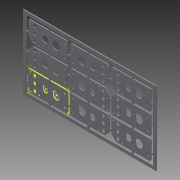
# Autodesk Inventor part: Granny Gearbox Output Plate Routing Template (9-up)
Saved by Autodesk Inventor 2015 (Build 190159000, 159)
## iProperties
Created: 2016-02-25
Part Number: Granny Gearbox Output Plate Routing Template (9-up)
Material: Generic
Document SubType Name: Modeling
Designer: sethbattis
Density: 1 g/cm^3
Appearance: Default
Author: sethbattis
Autodesk Inventor part; units mm, degrees
ref_plane "YZ Plane" through (0, 0, 0) normal (1, 0, 0) x (0, 1, 0)
ref_plane "XZ Plane" through (0, 0, 0) normal (0, 1, 0) x (-1, 0, 0)
ref_plane "XY Plane" through (0, 0, 0) normal (0, 0, 1) x (1, 0, 0)
derived "Granny Gearbox Output Plate.ipt"
sketch "New Mounting Holes" plane through (0, 0, 0) normal (0, 0, 1) x (1, 0, 0)
  circle A0 centre (74.3367, 23.3553) radius 3.175
  circle A1 centre (74.3367, -23.3553) radius 3.175
  circle A2 centre (-57.7242, 30.4609) radius 3.175
  circle A3 centre (-24.3812, -30.912) radius 3.175
  line L0 (-65.3633, -38.1) -> (-65.3633, 38.1) construction
  line L1 (87.0367, -38.1) -> (-65.3633, -38.1) construction
  line L2 (87.0367, 38.1) -> (87.0367, -38.1) construction
  line L3 (-65.3633, 38.1) -> (87.0367, 38.1) construction
  line L4 (-55.8383, 38.1) -> (-55.8383, -38.1) construction
  line L5 (-65.3633, 28.575) -> (87.0367, 28.575) construction
  line L6 (-65.3633, -28.575) -> (87.0367, -28.575) construction
  line L7 (77.5117, 38.1) -> (77.5117, -38.1) construction
  circle A4 centre (-40.7035, -0.0359) radius 31.75 construction
  circle A5 centre (40.6908, 0) radius 36.195 construction
  circle A6 centre (0, 0) radius 36.195 construction
  line L8 (-57.7242, 30.4609) -> (-55.8383, 30.4609) construction
  line L9 (-57.7242, 30.4609) -> (-57.7242, 28.575) construction
sketch "Labels" plane through (0, 0, 0) normal (0, 0, 1) x (1, 0, 0)
  circle A0 centre (-40.7035, -0.0359) radius 5.5626
  circle A1 centre (-40.7035, 25.3641) radius 5.5626
  circle A2 centre (-40.7035, -25.4359) radius 5.5626
  circle A3 centre (0, 0) radius 11.1125
  circle A4 centre (40.6908, 0) radius 14.2875
  line L0 (-5.8677, 26.2224) -> (48.5566, 26.2224) construction
  line L1 (48.5566, 26.2224) -> (48.5566, 22.1963) construction
  line L2 (48.5566, 22.1963) -> (-5.8677, 22.1963) construction
  line L3 (-5.8677, 22.1963) -> (-5.8677, 26.2224) construction
sketch "Exterior" plane through (0, 0, 0) normal (0, 0, 1) x (1, 0, 0)
  line L0 (-59.0133, 38.1) -> (80.6867, 38.1)
  line L1 (87.0367, 31.75) -> (87.0367, -31.75)
  line L2 (80.6867, -38.1) -> (-44.6678, -38.1)
  arc A0 (87.0367, 31.75) -> (80.6867, 38.1) centre (80.6867, 31.75) ccw
  arc A1 (80.6867, -38.1) -> (87.0367, -31.75) centre (80.6867, -31.75) ccw
  arc A2 (-59.0133, 38.1) -> (-65.3633, 31.75) centre (-59.0133, 31.75) ccw
  circle A3 centre (-40.7035, -0.0359) radius 31.75 construction
  line L3 (-65.3633, -17.4045) -> (-65.3633, 31.75)
  line L4 (-63.5034, -21.8946) -> (-49.1579, -36.2401)
  line L5 (-65.3633, -38.1) -> (-65.3633, 38.1) construction
  line L6 (87.0367, -38.1) -> (-65.3633, -38.1) construction
  arc A4 (-49.1579, -36.2401) -> (-44.6678, -38.1) centre (-44.6678, -31.75) ccw
  arc A5 (-65.3633, -17.4045) -> (-63.5034, -21.8946) centre (-59.0133, -17.4045) ccw
  point P0 (87.0367, 38.1)
  point P1 (-65.3633, -20.0348)
  point P2 (-47.2981, -38.1)
sketch "Sketch1" plane through (0, 0, 0) normal (0, 0, 1) x (1, 0, 0)
  circle A0 centre (-57.7242, 30.4609) radius 3.175 projected
  circle A1 centre (74.3367, 23.3553) radius 3.175 projected
  circle A2 centre (74.3367, -23.3553) radius 3.175 projected
  circle A3 centre (-24.3812, -30.912) radius 3.175 projected
  circle A4 centre (-40.7035, 25.3641) radius 6.3563
  circle A5 centre (-40.7035, -0.0359) radius 6.3563
  circle A6 centre (-40.7035, -25.4359) radius 6.3563
  circle A7 centre (0, 0) radius 11.9062
  circle A8 centre (40.6908, 0) radius 15.0812
  circle A9 centre (74.3367, 23.3553) radius 3.175
  circle A10 centre (74.3367, -23.3553) radius 3.175
  circle A11 centre (-24.3812, -30.912) radius 3.175
  circle A12 centre (-57.7242, 30.4609) radius 3.175
  circle A13 centre (-40.7035, -0.0359) radius 5.5626 projected
  circle A14 centre (-40.7035, -25.4359) radius 5.5626 projected
  circle A15 centre (-40.7035, 25.3641) radius 5.5626 projected
  circle A16 centre (0, 0) radius 11.1125 projected
  circle A17 centre (40.6908, 0) radius 14.2875 projected
  line L0 (-58.2195, 37.3062) -> (12.6355, 37.3062)
  line L1 (86.243, 30.9562) -> (86.243, -5.069)
  line L2 (79.893, -37.3063) -> (18.9865, -37.3062)
  line L3 (-65.3633, 38.1) -> (87.0367, 38.1) construction
  line L4 (87.0367, 38.1) -> (87.0367, -38.1) construction
  line L5 (87.0367, -38.1) -> (-65.3633, -38.1) construction
  line L6 (-63.5034, -21.8946) -> (-49.1579, -36.2401) projected
  line L7 (-65.3633, -38.1) -> (-65.3633, 38.1) construction
  line L8 (-62.7097, -21.5659) -> (-48.8291, -35.4464)
  line L9 (-64.5695, -17.0757) -> (-64.5695, -11.419)
  arc A18 (-58.2195, 37.3062) -> (-64.5695, 30.9562) centre (-58.2195, 30.9562) ccw
  arc A19 (-64.5695, -17.0757) -> (-62.7097, -21.5659) centre (-58.2195, -17.0757) ccw
  arc A20 (-48.8291, -35.4464) -> (-44.339, -37.3063) centre (-44.339, -30.9563) ccw
  arc A21 (79.893, -37.3063) -> (86.243, -30.9562) centre (79.893, -30.9562) ccw
  arc A22 (86.243, 30.9562) -> (79.893, 37.3062) centre (79.893, 30.9562) ccw
  line L10 (18.9855, 37.3062) -> (18.9855, 41.3004)
  line L11 (18.9855, 41.3004) -> (12.6355, 41.3004)
  line L12 (12.6355, 41.3004) -> (12.6355, 37.3062)
  line L13 (18.9865, -37.3062) -> (18.9854, -41.3004)
  line L14 (18.9854, -41.3004) -> (12.6344, -41.3004)
  line L15 (12.6344, -41.3004) -> (12.6354, -37.3062)
  line L16 (86.243, -11.419) -> (90.2371, -11.419)
  line L17 (90.2371, -11.419) -> (90.2371, -5.069)
  line L18 (90.2371, -5.069) -> (86.243, -5.069)
  line L19 (-64.5695, -11.419) -> (-68.5637, -11.419)
  line L20 (-68.5637, -11.419) -> (-68.5637, -5.069)
  line L21 (-68.5637, -5.069) -> (-64.5695, -5.069)
  line L22 (18.9855, 37.3062) -> (79.893, 37.3062)
  line L23 (86.243, -11.419) -> (86.243, -30.9562)
  line L24 (12.6354, -37.3062) -> (-44.339, -37.3063)
  line L25 (-64.5695, -5.069) -> (-64.5695, 30.9562)
  dimension "d15" = 0.7937
  dimension "d18" = 0.7937
  dimension "d19" = 0.7937
  dimension "d21" = 0.7937
  dimension "d22" = 6.35
  dimension "d23" = 28.575
  dimension "d24" = 30.1625
  dimension "d25" = 22.225
  dimension "d26" = 23.8125
  dimension "d27" = 11.1252
  dimension "d28" = 12.7127
  dimension "d31" = 6.35
  dimension "d34" = 3.9942
  dimension "d57" = 0.7937
  constraints: 42 end point, 18 tangent, 14 centre point, 13 parallel, 10 equal radius, 10 point on circle, 9 coincident, 6 horizontal, 6 perpendicular, 5 concentric, 5 equal length, 4 point on line, 1 collinear
  measures "d15" distance between parallel lines of L0 L3
  measures "d18" distance between parallel lines of L1 L4
  measures "d19" distance between parallel lines of L5 L2
  measures "d21" distance between parallel lines of L8 L6
  measures "d22" radius of A18
  measures "d23" diameter of A17
  measures "d24" diameter of A8
  measures "d25" diameter of A16
  measures "d26" diameter of A7
  measures "d27" diameter of A15
  measures "d28" diameter of A4
  measures "d31" distance of L11.end L10.end
  measures "d34" distance of L10.start L10.end
  measures "d57" distance between parallel lines of L7 L25
extrude "Extrusion1" add sketch "Sketch1" along normal blind 3.175 contours L0 L12 L11 L10 L22 A22 L1 L18 L17 L16 L23 A21 L2 L13 L14 L15 L24 A20 L8 A19 L9 L19 L20 L21 L25 A18
mirror "Mirror1" about plane through (90.2371, -11.419, 0) normal (1, 0, 0)
mirror "Mirror2" about plane through (249.0379, -5.069, 0) normal (1, 0, 0) of "Mirror1"
mirror "Mirror3" about plane through (161.4888, 41.3004, 0) normal (0, 1, 0)
mirror "Mirror4" about plane through (330.236, 123.9012, 0) normal (0, 1, 0) of "Mirror3"
sketch "Sketch5" plane through (0, 0, 0) normal (0, 0, 1) x (1, 0, 0)
  line L0 (-72.5578, 210.4961) -> (-72.5578, 160.1326)
  line L1 (-72.5578, -45.2945) -> (-85.2578, -45.2945)
  line L2 (-85.2578, -45.2945) -> (-85.2578, 200.5697)
  line L3 (411.8329, 210.4961) -> (411.8329, 223.1961)
  line L4 (411.8329, 223.1961) -> (-85.2578, 223.1961)
  line L5 (-85.2578, 223.1961) -> (-85.2578, 200.5697)
  line L6 (-72.5578, 210.4961) -> (12.6355, 210.4961)
  line L7 (-44.339, -37.3063) -> (12.6354, -37.3062) projected
  line L8 (407.8387, 153.7826) -> (407.8387, 160.1326) projected
  line L9 (12.6344, -41.3004) -> (18.9854, -41.3004) projected
  line L10 (12.6355, 206.502) -> (18.9855, 206.502)
  line L11 (18.9855, 206.502) -> (18.9855, 210.4961)
  line L12 (12.6355, 210.4961) -> (12.6355, 206.502)
  line L13 (161.4888, 206.502) -> (167.8367, 206.502)
  line L14 (167.8367, 206.502) -> (167.8367, 210.4961)
  line L15 (161.4888, 210.4961) -> (161.4888, 206.502)
  line L16 (330.2371, 206.502) -> (336.5871, 206.502)
  line L17 (336.5871, 206.502) -> (336.5871, 210.4961)
  line L18 (330.2371, 210.4961) -> (330.2371, 206.502)
  line L19 (-68.5637, 160.1326) -> (-72.5578, 160.1326)
  line L20 (-72.5578, 153.7826) -> (-68.5637, 153.7826)
  line L21 (-68.5637, 153.7826) -> (-68.5637, 160.1326)
  line L22 (-68.5637, 160.1326) -> (-68.5637, 153.7826) projected
  line L23 (-68.5637, 94.0198) -> (-72.5578, 94.0198)
  line L24 (-72.5578, 87.6698) -> (-68.5637, 87.6698)
  line L25 (-68.5637, 87.6698) -> (-68.5637, 94.0198)
  line L26 (-68.5637, -5.069) -> (-72.5578, -5.069)
  line L27 (-72.5578, -11.419) -> (-68.5637, -11.419)
  line L28 (-68.5637, -11.419) -> (-68.5637, -5.069)
  line L29 (-72.5578, -11.419) -> (-72.5578, -45.2945)
  line L30 (-72.5578, 87.6698) -> (-72.5578, -5.069)
  line L31 (-72.5578, 153.7826) -> (-72.5578, 94.0198)
  line L32 (18.9855, 210.4961) -> (161.4888, 210.4961)
  line L33 (167.8367, 210.4961) -> (330.2371, 210.4961)
  line L34 (336.5871, 210.4961) -> (411.8329, 210.4961)
  point P0 (0, 0)
  dimension "d38" = 3.9942
  dimension "d39" = 3.9942
  dimension "d42" = 12.7
  dimension "d44" = 12.7
  dimension "d51" = 3.9942
  dimension "d52" = 3.9942
  constraints: 62 end point, 14 parallel, 11 horizontal, 9 point on line, 3 perpendicular, 1 collinear, 1 vertical
  measures "d38" distance between parallel lines of L6 L16
  measures "d39" distance between parallel lines of L22 L0
  measures "d42" distance between parallel lines of L4 L34
  measures "d44" distance between parallel lines of L2 L29
  measures "d51" distance between parallel lines of L9 L1
  measures "d52" distance between parallel lines of L3 L8
extrude "Extrusion2" add sketch "Sketch5" along normal blind 3.175
sketch "Sketch7" plane through (0, 0, 0) normal (0, 0, 1) x (1, 0, 0)
  line L0 (-85.2578, -57.9945) -> (424.5329, -57.9945)
  line L1 (411.8329, -45.2945) -> (336.586, -45.2945)
  line L2 (-85.2578, -45.2945) -> (-85.2578, -57.9945)
  line L3 (-85.2578, 223.1961) -> (-85.2578, -45.2945) projected
  line L4 (12.6344, -41.3004) -> (18.9854, -41.3004) projected
  line L5 (411.8329, 223.1961) -> (-85.2578, 223.1961) projected
  line L6 (411.8329, 223.1961) -> (424.5329, 223.1961)
  line L7 (424.5329, 223.1961) -> (424.5329, -59.4551)
  line L8 (336.587, -41.3004) -> (330.236, -41.3004)
  line L9 (330.236, -41.3004) -> (330.2349, -45.2945)
  line L10 (336.586, -45.2945) -> (336.587, -41.3004)
  line L11 (161.4888, -41.3004) -> (167.8398, -41.3004)
  line L12 (167.8398, -41.3004) -> (167.8409, -45.2945)
  line L13 (161.4898, -45.2945) -> (161.4888, -41.3004)
  line L14 (12.6344, -41.3004) -> (18.9865, -41.3004)
  line L15 (18.9865, -41.3004) -> (18.9865, -45.2945)
  line L16 (12.6344, -45.2945) -> (12.6344, -41.3004)
  line L17 (407.8387, 160.1326) -> (411.8329, 160.1326)
  line L18 (411.8329, 153.7826) -> (407.8387, 153.7826)
  line L19 (407.8387, -5.069) -> (411.8329, -5.069)
  line L20 (411.8329, -11.419) -> (407.8387, -11.419)
  line L21 (12.6344, -45.2945) -> (-85.2578, -45.2945)
  line L22 (161.4898, -45.2945) -> (18.9865, -45.2945)
  line L23 (330.2349, -45.2945) -> (167.8409, -45.2945)
  line L24 (411.8329, -5.069) -> (411.8329, 86.9395)
  line L25 (411.8329, 93.2895) -> (411.8329, 153.7826)
  line L26 (411.8329, 160.1326) -> (411.8329, 223.1961)
  line L27 (411.8329, -45.2945) -> (411.8329, -11.419)
  line L28 (167.8388, -37.3062) -> (167.8398, -41.3004) projected
  line L29 (167.8398, -41.3004) -> (161.4888, -41.3004) projected
  line L30 (18.9854, -41.3004) -> (18.9865, -37.3062) projected
  line L31 (330.237, -37.3062) -> (330.236, -41.3004) projected
  line L32 (403.8446, -11.419) -> (407.8387, -11.419) projected
  line L33 (407.8387, -5.069) -> (407.8387, -11.419)
  line L34 (407.8387, -11.419) -> (407.8387, -5.069) projected
  line L35 (403.8446, 153.7826) -> (407.8387, 153.7826) projected
  line L36 (407.8387, 160.1326) -> (407.8387, 153.7826)
  line L37 (407.8387, 153.7826) -> (407.8387, 160.1326) projected
  line L38 (411.8329, 210.4961) -> (411.8329, 223.1961) projected
  line L39 (-85.2578, -45.2945) -> (-72.5578, -45.2945) projected
  line L40 (411.8329, 93.2895) -> (407.1085, 93.2895)
  line L41 (407.1085, 93.2895) -> (407.1085, 86.9395)
  line L42 (407.1085, 86.9395) -> (411.8329, 86.9395)
  point P0 (0, 0)
  dimension "d53" = 12.7
  dimension "d54" = 12.7
  constraints: 60 end point, 15 collinear, 13 parallel, 8 horizontal, 4 perpendicular, 3 point on line, 1 equal length, 2 other
  measures "d53" distance between parallel lines of L0 L23
  measures "d54" distance between parallel lines of L27 L7
extrude "Extrusion3" add sketch "Sketch7" along normal blind 3.175 contours L2 L21 L16 L4 L15 L22 L13 L11 L12 L23 L9 L8 L10 L1 L27 L20 L33 L19 L24 L42 L41 L40 L25 L18 L36 L17 L26 L6 L7 L0
equation "\"d18\" = d15"
equation "\"d19\" = d15"
equation "\"d21\" = d15"
equation "\"d24\" = d23 + 2 * d15"
equation "\"d26\" = d25 + 2 * d15"
equation "\"d28\" = d27 + 2 * d15"
equation "\"d57\" = d15"
equation "\"d38\" = d34"
equation "\"d39\" = d34"
equation "\"d51\" = d34"
equation "\"d52\" = d34"
body "Solid2"
